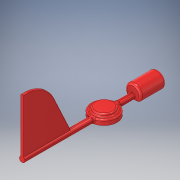
# Autodesk Inventor part: Direccion
Saved by Autodesk Inventor 2019 (Build 230136000, 136)
## iProperties
Created: 2019-12-17
Part Number: Direccion
Material: Generic
Document SubType Name: Modeling
Designer: Sergio
Density: 1 g/cm^3
Appearance: Light Red
Author: Sergio
Autodesk Inventor part; units mm, degrees
ref_plane "YZ Plane" through (0, 0, 0) normal (1, 0, 0) x (0, 1, 0)
ref_plane "XZ Plane" through (0, 0, 0) normal (0, 1, 0) x (-1, 0, 0)
ref_plane "XY Plane" through (0, 0, 0) normal (0, 0, 1) x (1, 0, 0)
sketch "Sketch1" plane through (0, 0, 0) normal (0, 1, 0) x (-1, 0, 0)
  line L0 (-4, -107.5) -> (4, -107.5)
  line L1 (4, 107.5) -> (-4, 107.5)
  line L2 (-4, -107.5) -> (4, 107.5) construction
  line L3 (4, -107.5) -> (-4, 107.5) construction
  line L4 (-4, 107.5) -> (-4, -2.2881)
  line L5 (-4, -42.5) -> (-4, -107.5)
  line L6 (4, -107.5) -> (4, -42.5)
  line L7 (4, -2.2881) -> (4, 107.5)
  arc A0 (4, -42.5) -> (4, -2.2881) centre (0, -22.394) ccw
  arc A1 (-4, -2.2881) -> (-4, -42.5) centre (0, -22.394) ccw
  point P0 (0, 0)
  dimension "d0" = 8
  dimension "d1" = 215
  dimension "d14" = 20.5
  dimension "d15" = 20.5
  dimension "d16" = 8
  dimension "d17" = 65
  constraints: 16 end point, 7 parallel, 4 point on circle, 2 centre point, 2 midpoint, 2 perpendicular, 1 horizontal
  measures "d0" distance of L1.end L1.start
  measures "d1" distance of L1.start L0.end
  measures "d14" radius of A0
  measures "d15" radius of A1
  measures "d16" distance between parallel lines of L5 L6
  measures "d17" distance of L5.start L0.start
extrude "Extrusion1" add sketch "Sketch1" along normal blind 8
sketch "Sketch2" plane through (0, 0, 0) normal (1, 0, 0) x (0, 1, 0)
  line L0 (8, 107.5) -> (8, 32.5)
  line L1 (8, 32.5) -> (64.2504, 58.73)
  line L2 (8, 107.5) -> (93, 107.5)
  arc A0 (64.2504, 58.73) -> (93, 107.5) centre (43.1195, 104.0454) ccw
  point P0 (0, 0)
  dimension "d6" = 75
  dimension "d7" = 85
  dimension "d9" = 65
  dimension "d11" = 50
  constraints: 6 end point, 2 point on circle, 1 centre point, 1 horizontal, 1 tangent
  measures "d6" distance of L0.start L0.end
  measures "d7" distance of L0.start L2.end
  measures "d9" angle of L0 L1
  measures "d11" radius of A0
extrude "Extrusion2" add sketch "Sketch2" along normal mid plane 4
sketch "Sketch4" plane through (4, 0, -107.5) normal (0, 0, -1) x (-1, 0, 0)
  arc A0 (13.1047, 0) -> (-6.1047, 0) centre (3.5, 8) ccw
  line L0 (0, 8) -> (8, 8) projected
  line L1 (8, 0) -> (8, 8) projected
  line L2 (-6.1047, 0) -> (13.1047, 0)
  line L3 (0, 0) -> (-16.5, 0) projected
  point P0 (4, 0)
  point P1 (0, 0)
  dimension "d19" = 25
  dimension "d20" = 0
  dimension "d21" = 4.5
  dimension "d76" = 0
  constraints: 2 end point, 2 point on circle, 1 centre point, 1 horizontal
  measures "d19" diameter of A0
  measures "d20" distance from line of L0 A0.centre
  measures "d21" distance from line of L1 A0.centre
  measures "d76" distance between parallel lines of L3 L2
extrude "Extrusion3" add sketch "Sketch4" against normal blind 40
fillet "Fillet2" radius 0.8 2 edges at (-2, 86.1925, 78.6541) (-2, 36.1252, 45.615)
fillet "Fillet3" radius 0.8 2 edges at (2, 86.1925, 78.6541) (2, 36.1252, 45.615)
sketch "Sketch5" plane through (0, 0, 0) normal (0, -1, 0) x (1, 0, 0)
  circle A0 centre (0, -22.394) radius 12.5
  arc A1 (-4, -2.2881) -> (-4, -42.5) centre (0, -22.394) ccw projected
  point P0 (0, 0)
  dimension "d27" = 25
  constraints: 1 centre point, 1 concentric
  measures "d27" diameter of A0
extrude "Extrusion4" cut sketch "Sketch5" against normal blind 7
sketch "Sketch10" plane through (0, 8, 0) normal (0, 1, 0) x (1, 0, 0)
  circle A0 centre (0, 22.394) radius 20.5
  circle A1 centre (0, 22.394) radius 12.5 projected
  point P0 (0, 0)
  point P1 (0, 1.0521)
  dimension "d53" = 41
  constraints: 1 centre point, 1 concentric
  measures "d53" diameter of A0
extrude "Extrusion6" add sketch "Sketch10" along normal blind 4 contours A0 | A1
sketch "Sketch11" plane through (0, 12, -22.394) normal (0, 1, 0) x (1, 0, 0)
  circle A0 centre (0, 0) radius 20.5
  circle A1 centre (0, 0) radius 15
  circle A2 centre (0, 0) radius 20.5 projected
  point P0 (0, -22.394)
  dimension "d57" = 41
  dimension "d58" = 30
  constraints: 2 centre point, 1 concentric
  measures "d57" diameter of A0
  measures "d58" diameter of A1
extrude "Extrusion7" cut sketch "Sketch11" against normal blind 4
fillet "Fillet14" radius 3 8 edges at (4, 8, 52.606) (-4, 8, 52.606) (4, 8, -55) (-4, 8, -55) (-4, 0, 52.606) (4, 0, 52.606) (-4, 0, -55) (4, 0, -55)
fillet "Fillet15" radius 3 4 edges at (0.5, 20.5, -107.5) (0.5, 20.5, -67.5) (10.1047, 0, -87.5) (-9.1047, 0, -87.5)
fillet "Fillet16" radius 2 4 edges at (4, 4, -2.2881) (-4, 4, -2.2881) (4, 4, -42.5) (-4, 4, -42.5)
sketch "Sketch14" plane through (0, 0, 0) normal (0, -1, 0) x (1, 0, 0)
  circle A0 centre (0, -22.394) radius 12.5
  circle A1 centre (0, -22.394) radius 12.5 projected
  circle A2 centre (0, -22.394) radius 20.5
  arc A3 (4.5556, -42.3814) -> (4.5556, -2.4066) centre (0, -22.394) ccw projected
  point P0 (0, 0)
  constraints: 4 concentric, 2 centre point
fillet "Fillet17" radius 2 7 edges at (-15, 12, -22.394) (-15, 8, -22.394) (2.7158, 8, -43.336) (2.7158, 8, -1.4521) (-2.7158, 8, -43.336) (-2.7158, 8, -1.4521) (20.5, 8, -22.394)
body "Solid1"
